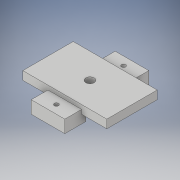
# Autodesk Inventor part: mount
Saved by Autodesk Inventor 2017 (Build 210142000, 142)
## iProperties
Created: 2017-03-20
Part Number: mount
Material: Generic
Document SubType Name: Modeling
Designer: Naga
Density: 1 g/cm^3
Appearance: Default
Author: Naga
Autodesk Inventor part; units mm, degrees
ref_plane "YZ Plane" through (0, 0, 0) normal (1, 0, 0) x (0, 1, 0)
ref_plane "XZ Plane" through (0, 0, 0) normal (0, 1, 0) x (-1, 0, 0)
ref_plane "XY Plane" through (0, 0, 0) normal (0, 0, 1) x (1, 0, 0)
sketch "Sketch1" plane through (0, 0, 0) normal (0, 1, 0) x (-1, 0, 0)
  line L0 (0, 0) -> (63.5, 0)
  line L1 (63.5, 0) -> (63.5, -38.1)
  line L2 (63.5, -38.1) -> (0, -38.1)
  line L3 (0, -38.1) -> (0, 0)
  dimension "d0" = 63.5
  dimension "d1" = 38.1
  constraints: 8 end point, 2 parallel, 1 horizontal, 1 perpendicular
  measures "d0" distance of L1.end L2.end
  measures "d1" distance of L0.end L1.end
extrude "Extrusion1" add sketch "Sketch1" along normal blind 6.35
sketch "Sketch2" plane through (0, 6.35, 0) normal (0, 1, 0) x (1, 0, 0)
  line L0 (-63.5, 0) -> (0, 0) projected
  line L1 (0, 0) -> (0, 38.1) projected
  line L2 (0, 38.1) -> (-63.5, 38.1) projected
  line L3 (-63.5, 38.1) -> (-63.5, 0) projected
  line L4 (0, 0) -> (0, 38.1) construction
  line L5 (0, 19.05) -> (-31.75, 19.05) construction
  circle A0 centre (-31.75, 19.05) radius 3.175
  dimension "d4" = 31.75
  dimension "d5" = 90
  dimension "d6" = 6.35
  constraints: 2 end point, 1 centre point, 1 coincident, 1 midpoint
  measures "d4" distance of L5.start L5.end
  measures "d5" angle of L5 L1
  measures "d6" diameter of A0
extrude "Extrusion2" cut sketch "Sketch2" against normal blind 6.35 contours A0
sketch "Sketch3" plane through (0, 0, 0) normal (0, -1, 0) x (1, 0, 0)
  circle A0 centre (-31.75, -19.05) radius 3.175 projected
  line L0 (0, 0) -> (-63.5, 0) projected
  line L1 (-63.5, 0) -> (-63.5, -38.1) projected
  line L2 (-63.5, -38.1) -> (0, -38.1) projected
  line L3 (0, -38.1) -> (0, 0) projected
  line L4 (-31.75, -19.05) -> (-19.05, -19.05) construction
  line L5 (-19.05, -19.05) -> (-19.05, 12.7) construction
  line L6 (-19.05, 12.7) -> (-19.05, -50.8) construction
  line L7 (-19.05, 12.7) -> (-44.45, 12.7)
  line L8 (-44.45, 12.7) -> (-44.45, -3.175)
  line L9 (-44.45, -3.175) -> (-19.05, -3.175)
  line L10 (-19.05, -3.175) -> (-19.05, 12.7)
  circle A1 centre (-31.75, -19.05) radius 3.175 construction
  line L11 (-31.75, -19.05) -> (-31.75, 6.35) construction
  line L12 (-31.75, -19.05) -> (-6.35, -19.05) construction
  circle A2 centre (-31.75, 6.35) radius 1.5875
  line L13 (-19.05, -19.05) -> (-19.05, -50.8) construction
  line L14 (-19.05, -50.8) -> (-19.05, 12.7) construction
  line L15 (-19.05, -50.8) -> (-44.45, -50.8)
  line L16 (-44.45, -50.8) -> (-44.45, -34.925)
  line L17 (-44.45, -34.925) -> (-19.05, -34.925)
  line L18 (-19.05, -34.925) -> (-19.05, -50.8)
  circle A3 centre (-31.75, -44.45) radius 1.5875
  dimension "d9" = 12.7
  dimension "d10" = 31.75
  dimension "d11" = 63.5
  dimension "d12" = 25.4
  dimension "d13" = 15.875
  dimension "d14" = 25.4
  dimension "d15" = 90
  dimension "d16" = 3.175
  constraints: 30 end point, 7 symmetric about line, 3 horizontal, 3 perpendicular, 2 centre point, 2 coincident, 2 parallel, 2 point on line, 1 vertical, 1 other
  measures "d9" distance of L4.start L4.end
  measures "d10" distance of L4.end L5.end
  measures "d11" distance of L5.end L6.end
  measures "d12" distance of L9.end L8.end
  measures "d13" distance of L8.end L7.end
  measures "d14" distance of L11.start L11.end
  measures "d15" angle of L12 L11
  measures "d16" diameter of A2
extrude "Extrusion3" add sketch "Sketch3" along normal blind 6.35 and the other way blind 3.175 contours L10 L9 L8 L0 | L0 L8 L7 L10 | L18 L15 L16 L2 | L2 L16 L17 L18
body "Solid1"
